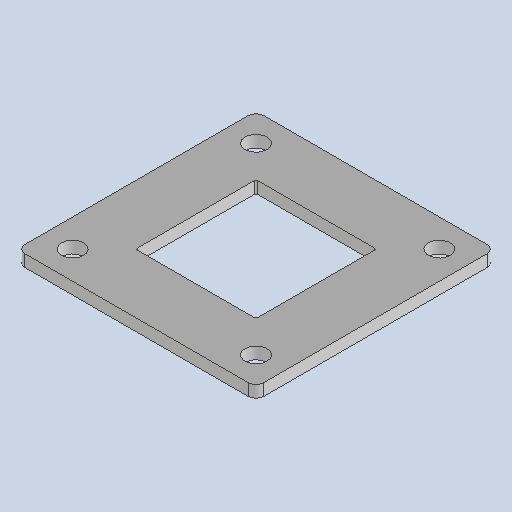
# Autodesk Inventor part: PRS 1425 DrSysB Way FLANGE_1200
Saved by Autodesk Inventor 2026.2 (Build 302298000, 298)
## iProperties
Created: 2025-06-24
Part Number: PRS 1425 DrSysB Way FLANGE_1200
Material: Stainless Steel
Document SubType Name: Sheet Metal
Designer: admin
Mass: 62.1684 g
Surface Area: 64.55 cm^2
Volume: 7.77105 cm^3
Density: 8 g/cm^3
Flat Pattern Width: 6 cm
Flat Pattern Length: 6 cm
Flat Pattern Area: 36 cm^2
Sheet Metal Rule: AISI304 2mm Die16
Sheet Metal Width: 60,000 mm
Sheet Metal Length: 60,000 mm
Sheet Metal Area: 3600,000 mm^2
Appearance: Default
Author: user
Autodesk Inventor part; units mm, degrees
ref_plane "YZ Plane" through (0, 0, 0) normal (1, 0, 0) x (0, 1, 0)
ref_plane "XZ Plane" through (0, 0, 0) normal (0, 1, 0) x (-1, 0, 0)
ref_plane "XY Plane" through (0, 0, 0) normal (0, 0, 1) x (1, 0, 0)
sketch "Sketch1" plane through (0, 0, 0) normal (0, 0, 1) x (1, 0, 0)
  line L0 (-30, -30) -> (30, -30)
  line L1 (30, -30) -> (30, 30)
  line L2 (30, 30) -> (-30, 30)
  line L3 (-30, 30) -> (-30, -30)
  line L4 (-30, -30) -> (30, 30) construction
  line L5 (30, -30) -> (-30, 30) construction
  line L6 (15.1, -15.1) -> (-15.1, -15.1)
  line L7 (-15.1, -15.1) -> (-15.1, 15.1)
  line L8 (-15.1, 15.1) -> (15.1, 15.1)
  line L9 (15.1, 15.1) -> (15.1, -15.1)
  line L10 (15.1, -15.1) -> (-15.1, 15.1) construction
  line L11 (-15.1, -15.1) -> (15.1, 15.1) construction
  circle A0 centre (-23, -23) radius 2.75
  circle A1 centre (23, -23) radius 2.75
  circle A2 centre (23, 23) radius 2.75
  circle A3 centre (-23, 23) radius 2.75
  line L12 (25.75, 25.75) -> (-25.75, 25.75) construction
  line L13 (-25.75, 25.75) -> (-25.75, -25.75) construction
  line L14 (-25.75, -25.75) -> (25.75, -25.75) construction
  line L15 (25.75, -25.75) -> (25.75, 25.75) construction
  line L16 (25.75, 25.75) -> (-25.75, -25.75) construction
  line L17 (-25.75, 25.75) -> (25.75, -25.75) construction
  line L18 (23, 23) -> (-23, 23) construction
  line L19 (-23, 23) -> (-23, -23) construction
  line L20 (-23, -23) -> (23, -23) construction
  line L21 (23, -23) -> (23, 23) construction
  line L22 (23, 23) -> (-23, -23) construction
  line L23 (-23, 23) -> (23, -23) construction
  point P0 (0, 0)
  dimension "d172" = 30.2
  dimension "d190" = 5.5
  dimension "d191" = 46
  dimension "d192" = 60
  measures "d172" distance of L7.end L8.end
  measures "d190" diameter of A0
  measures "d191" distance of L19.end L20.end
  measures "d192" distance of L2.end L0.start
extrude "Plate5" add sketch "Sketch1" along normal blind 3
fillet "Corner Round1" radius 2 4 edges at (30, 30, 1.5) (-30, 30, 1.5) (-30, -30, 1.5) (30, -30, 1.5)
fillet "Corner Round2" radius 0.5 4 edges at (-15.1, 15.1, 1.5) (-15.1, -15.1, 1.5) (15.1, -15.1, 1.5) (15.1, 15.1, 1.5)
body "Solid3"
